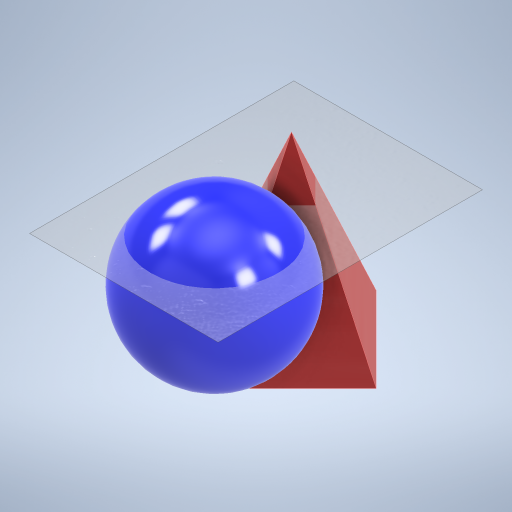
# Autodesk Inventor part: а
Saved by Autodesk Inventor 2024.2 (Build 282272000, 272)
## iProperties
Created: 2024-10-31
Part Number: а
Material: Типовые
Document SubType Name: Modeling
Designer: user
Density: 1 g/cm^3
Appearance: Красный
Mass: 519.616 g
Surface Area: 725.566 cm^2
Volume: 519.616 cm^3
Author: user
Autodesk Inventor part; units mm, degrees
ref_plane "YZ Plane" through (0, 0, 0) normal (1, 0, 0) x (0, 1, 0)
ref_plane "XY Plane" through (0, 0, 0) normal (0, 0, 1) x (1, 0, 0)
sketch "Эскиз1" plane through (0, 0, 0) normal (0, 0, 1) x (1, 0, 0)
  point P0 (0, 0)
sketch "Эскиз2" plane through (0, 0, 0) normal (1, 0, 0) x (0, 1, 0)
  circle A0 centre (50, 0) radius 45
  line L0 (5, 0) -> (95, 0)
  point P0 (0, 0)
  constraints: 2 end point, 2 point on circle, 1 centre point
revolve "Вращение1" add sketch "Эскиз2" angle 360 about axis through (0, 5, 0) along (0, 1, 0) picked at (45.3647, -14.2658) contours A0 L0
sketch "Эскиз3" plane through (0, 0, 0) normal (0, 1, 0) x (-1, 0, 0)
  line L0 (0, 4.4975) -> (49.4975, -45)
  line L1 (49.4975, -45) -> (0, -94.4975)
  line L2 (0, -94.4975) -> (-49.4975, -45)
  line L3 (-49.4975, -45) -> (0, 4.4975)
  point P0 (0, 0)
  point P1 (0, -45)
  constraints: 8 end point, 9 other
ref_plane "РабПлоскость2" through (0, 105, 0) normal (0, 1, 0) x (-1, 0, 0)
ref_plane "РабПлоскость1" through (0, 75, 0) normal (0, 1, 0) x (-1, 0, 0)
sketch "Эскиз4" plane through (0, 105, 0) normal (0, 1, 0) x (-1, 0, 0)
  point P0 (0, 0)
  point P1 (0, -45)
loft "Лофт1" add profiles "Эскиз3" section 1 point at (0, 105, -45)
sketch "Эскиз6" plane through (0, 75, 0) normal (0, 1, 0) x (-1, 0, 0)
  point P0 (0, 0)
sketch "Эскиз8" plane through (0, 75, 0) normal (0, 1, 0) x (-1, 0, 0)
  line L0 (55.196, -101.5768) -> (-54.9247, -101.5768)
  line L1 (-54.9247, -101.5768) -> (-54.9247, 52.7549)
  line L2 (-54.9247, 52.7549) -> (55.196, 52.7549)
  line L3 (55.196, 52.7549) -> (55.196, -101.5768)
  point P0 (0, 0)
  constraints: 8 end point, 3 perpendicular, 1 horizontal
extrude "Выдавливание3" add sketch "Эскиз8" against normal blind 0.1 separate body
